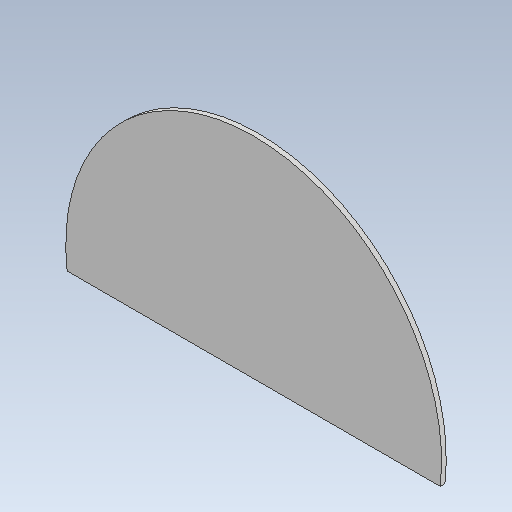
# Autodesk Inventor part: cover_side
Saved by Autodesk Inventor 2021 (Build 250183000, 183)
## iProperties
Created: 2021-05-06
Part Number: cover_side
Material: Generic
Document SubType Name: Modeling
Designer: Watchdog
Density: 1 g/cm^3
Appearance: Default
Author: Watchdog
Autodesk Inventor part; units mm, degrees
ref_plane "YZ Plane" through (0, 0, 0) normal (1, 0, 0) x (0, 1, 0)
ref_plane "XZ Plane" through (0, 0, 0) normal (0, 1, 0) x (-1, 0, 0)
ref_plane "XY Plane" through (0, 0, 0) normal (0, 0, 1) x (1, 0, 0)
sketch "Sketch2" plane through (0, 0, 0) normal (0, 0, 1) x (1, 0, 0)
  arc A0 (790, 0) -> (-790, 0) centre (0, 94.382) ccw
  line L0 (-790, 0) -> (790, 0)
  point P0 (0, 0)
  point P1 (0, 890)
  dimension "d17" = 0
  dimension "d21" = 0
  dimension "d24" = 890
  dimension "d25" = 1580
  dimension "d26" = 790
  constraints: 3 point on circle, 2 end point, 1 centre point, 1 horizontal
  measures "d17" horizontal distance of point (0, 0) point (0, 890)
  measures "d21" vertical distance of point (0, 0) L0.start
  measures "d24" distance of point (0, 0) point (0, 890)
  measures "d25" distance of L0.end L0.start
  measures "d26" distance of point (0, 0) L0.start
extrude "side" add sketch "Sketch2" along normal blind 20
equation "\"d24\" = cover_height_main - cover_shell_thickness"
equation "\"d25\" = cover_length_main - 2 * cover_shell_thickness"
equation "\"d26\" = 0.5 * d25"
equation "\"d14\" = cover_side_thickness"
equation "\"cover_height_main\" = 900"
equation "\"cover_shell_thickness\" = 10"
equation "\"cover_side_thickness\" = 20"
equation "\"hoop_angle_z\" = 45deg"
equation "\"hoop_bearing_length\" = 5deg"
equation "\"hoop_cable_diam\" = 5"
equation "\"hoop_cable_pulley_diam\" = 22"
equation "\"rack_tooth_addendum\" = 5"
equation "\"rack_tooth_dedendum\" = 5"
equation "\"rack_tooth_thickness\" = 5"
equation "\"secure_arm_angle\" = 20deg"
equation "\"secure_arm_hold_length\" = 35"
equation "\"secure_arm_radii\" = 9"
equation "\"support_baseClamp_platformLengthBuffer\" = 35"
equation "\"support_baseClamp_platformThickness\" = 15"
equation "\"support_baseClamp_platformWidthBuffer\" = 0"
equation "\"support_baseClamp_sleeveHoleDiameter\" = 12"
equation "\"support_baseClamp_sleeveSweepTerminationAngle\" = 55deg"
equation "\"support_baseClamp_thickness\" = 8"
equation "\"support_frame_endHoleBuffer\" = 25"
equation "\"support_frame_squareBarFillet\" = 2"
equation "\"support_frame_squareBarThickness\" = 5"
equation "\"hoop_tabs_hole\" = 4"
equation "\"hoop_tabs_thickness\" = 6"
equation "\"cover_length_main\" = 1600"
body "Solid2"
